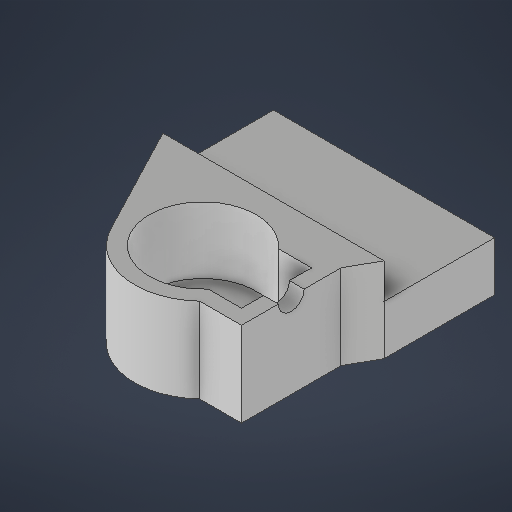
# Autodesk Inventor part: pitch_motor_standoff_v1
Saved by Autodesk Inventor 2026.2 (Build 302298000, 298)
## iProperties
Created: 2026-01-14
Part Number: pitch_motor_standoff_v1
Material: Generic
Document SubType Name: Modeling
Designer: User
Density: 1 g/cm^3
Appearance: Default
Author: User
Autodesk Inventor part; units mm, degrees
ref_plane "YZ Plane" through (0, 0, 0) normal (1, 0, 0) x (0, 1, 0)
ref_plane "XZ Plane" through (0, 0, 0) normal (0, 1, 0) x (-1, 0, 0)
ref_plane "XY Plane" through (0, 0, 0) normal (0, 0, 1) x (1, 0, 0)
sketch "Sketch1" plane through (0, 0, 0) normal (0, 1, 0) x (-1, 0, 0)
  arc A0 (-9.5, 10.9545) -> (9.5, 10.9545) centre (0, 0) ccw
  line L0 (-9.5, 10.9545) -> (-9.5, 20)
  line L1 (-9.5, 20) -> (9.5, 20)
  line L2 (9.5, 20) -> (9.5, 10.9545)
  line L3 (13.5, 12.6491) -> (13.5, 24)
  line L4 (13.5, 24) -> (-13.5, 24)
  line L5 (-13.5, 24) -> (-13.5, 12.6491)
  arc A1 (-13.5, 12.6491) -> (13.5, 12.6491) centre (0, 0) ccw
  point P0 (0, -20)
  point P1 (-9.5, 15)
  dimension "d0" = 0
  dimension "d1" = 29
  dimension "d6" = 20
  dimension "d7" = 19
  dimension "d8" = 4
  constraints: 12 end point, 4 point on circle, 2 centre point, 2 parallel, 1 coincident, 1 point on line, 3 other
  measures "d0" horizontal distance of A0.centre point (0, -20)
  measures "d1" diameter of A0
  measures "d6" distance from line of L1 point (0, 0)
  measures "d7" distance of L0.end L1.end
  measures "d8" radial gap between concentric circles of A0 A1
extrude "Extrusion1" add sketch "Sketch1" along normal blind 18
sketch "Sketch2" plane through (0, 18, 0) normal (0, 1, 0) x (1, 0, 0)
  arc A0 (13.5, -12.6491) -> (-13.5, -12.6491) centre (0, 0) ccw
  line L0 (-13.5, -12.6491) -> (-13.5, -24) projected
  line L1 (-13.5, -24) -> (13.5, -24)
  line L2 (13.5, -24) -> (13.5, -12.6491)
  line L3 (-13.5, -12.6491) -> (-13.5, -24)
  constraints: 6 end point, 2 point on circle, 1 centre point, 1 coincident, 1 horizontal, 1 parallel, 1 perpendicular
extrude "Extrusion2" add sketch "Sketch2" along normal blind 5
sketch "Sketch3" plane through (-13.5, 0, 24) normal (0, 0, 1) x (1, 0, 0)
  circle A0 centre (13.5, 0) radius 3.5
  dimension "d13" = 7
  constraints: 1 centre point, 1 coincident
  measures "d13" diameter of A0
extrude "Extrusion3" cut sketch "Sketch3" against normal blind 5
sketch "Sketch4" plane through (0, 0, 0) normal (0, -1, 0) x (1, 0, 0)
  line L0 (0, 0) -> (-21, 0)
  line L1 (-21, -31.8183) -> (-51, -31.8183)
  line L2 (-51, -31.8183) -> (-51, 28.1817)
  line L3 (-51, 28.1817) -> (-21, 28.1817)
  line L4 (-21, 28.1817) -> (-21, -31.8183)
  line L5 (-13.5, 24) -> (13.5, 24) projected
  line L6 (-21, 28.1817) -> (-13.5, 24)
  line L7 (-21, -31.8183) -> (8.5554, -16.4029)
  arc A0 (-13.5, 12.6491) -> (13.5, 12.6491) centre (0, 0) ccw projected
  arc A1 (-13.5, 12.6491) -> (8.5554, -16.4029) centre (0, 0) ccw
  line L8 (-13.5, 12.6491) -> (-13.5, 24) projected
  line L9 (-13.5, 24) -> (-13.5, 12.6491)
  dimension "d19" = 21
  dimension "d20" = 30
  dimension "d21" = 60
  constraints: 16 end point, 3 point on circle, 2 horizontal, 2 parallel, 1 centre point, 1 coincident, 1 perpendicular, 1 tangent, 1 vertical
  measures "d19" distance of L0.start L0.end
  measures "d20" distance of L2.end L3.end
  measures "d21" distance of L1.end L2.end
extrude "Extrusion4" add sketch "Sketch4" against normal blind 23
sketch "Sketch6" plane through (-21, 0, -31.8183) normal (0, 0, -1) x (-1, 0, 0)
  line L0 (0, 0) -> (-29.5554, 0) projected
  line L1 (0, 0) -> (30.3611, 0)
  line L2 (30.3611, 0) -> (30.3611, 9.5813)
  line L3 (30.3611, 9.5813) -> (0, 9.5813)
  line L4 (0, 9.5813) -> (0, 0)
  point P0 (-21, 0)
  dimension "d26" = 9.5813
  constraints: 8 end point, 2 parallel, 1 horizontal, 1 perpendicular
  measures "d26" distance of L2.end L1.end
extrude "Extrusion5" cut sketch "Sketch6" against normal through all
body "Solid1"
